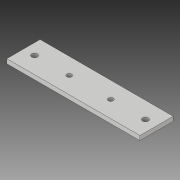
# Autodesk Inventor part: Manifold_Plate
Saved by Autodesk Inventor 2019 (Build 230136000, 136)
## iProperties
Created: 2021-08-02
Part Number: Manifold_Plate
Material: Generic
Document SubType Name: Modeling
Designer: devon
Density: 1 g/cm^3
Appearance: Default
Author: devon
Autodesk Inventor part; units mm, degrees
ref_plane "YZ Plane" through (0, 0, 0) normal (1, 0, 0) x (0, 1, 0)
ref_plane "XZ Plane" through (0, 0, 0) normal (0, 1, 0) x (-1, 0, 0)
ref_plane "XY Plane" through (0, 0, 0) normal (0, 0, 1) x (1, 0, 0)
sketch "Sketch1" plane through (0, 0, 0) normal (0, 1, 0) x (-1, 0, 0)
  line L0 (76.2, 19.05) -> (-76.2, 19.05)
  line L1 (-76.2, 19.05) -> (-76.2, -19.05)
  line L2 (-76.2, -19.05) -> (76.2, -19.05)
  line L3 (76.2, -19.05) -> (76.2, 19.05)
  line L4 (76.2, 19.05) -> (-76.2, -19.05) construction
  line L5 (-76.2, 19.05) -> (76.2, -19.05) construction
  point P0 (0, 0)
  dimension "d0" = 152.4
  dimension "d1" = 38.1
  constraints: 12 end point, 2 midpoint, 2 parallel, 1 horizontal, 1 perpendicular
  measures "d0" distance of L1.end L2.end
  measures "d1" distance of L2.end L0.start
extrude "Extrusion1" add sketch "Sketch1" along normal blind 5
sketch "Sketch2" plane through (0, 5, 0) normal (0, 1, 0) x (1, 0, 0)
  circle A0 centre (-23.8, 0) radius 2.75
  circle A1 centre (23.8, 0) radius 2.75
  circle A2 centre (-63.5, 0) radius 3.3
  circle A3 centre (63.5, 0) radius 3.3
  line L0 (-76.2, 19.05) -> (-76.2, -19.05) projected
  line L1 (76.2, -19.05) -> (76.2, 19.05) projected
  point P0 (0, 0)
  dimension "d4" = 5.5
  dimension "d5" = 5.5
  dimension "d6" = 47.6
  dimension "d7" = 23.8
  dimension "d8" = 6.6
  dimension "d9" = 6.6
  dimension "d10" = 12.7
  dimension "d11" = 12.7
  constraints: 4 centre point
  measures "d4" diameter of A0
  measures "d5" diameter of A1
  measures "d6" distance of A1.centre A0.centre
  measures "d7" distance of point (0, 0) A1.centre
  measures "d8" diameter of A2
  measures "d9" diameter of A3
  measures "d10" distance from line of L0 A2.centre
  measures "d11" distance from line of L1 A3.centre
extrude "Extrusion2" cut sketch "Sketch2" against normal up to next
body "Solid1"
